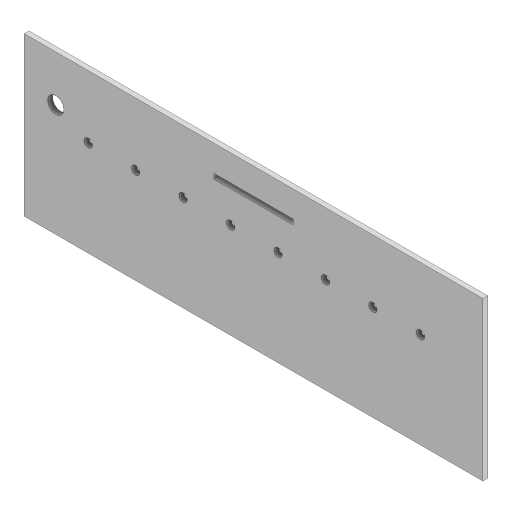
# Autodesk Inventor part: wall_ver.1
Saved by Autodesk Inventor 2024 (Build 280153000, 153)
## iProperties
Created: 2023-11-09
Part Number: wall_ver.1
Material: 一般
Document SubType Name: Modeling
Designer: moonshot
Density: 1 g/cm^3
Appearance: 既定
Author: moonshot
Autodesk Inventor part; units mm, degrees
ref_plane "YZ Plane" through (0, 0, 0) normal (1, 0, 0) x (0, 1, 0)
ref_plane "XZ Plane" through (0, 0, 0) normal (0, 1, 0) x (-1, 0, 0)
ref_plane "XY Plane" through (0, 0, 0) normal (0, 0, 1) x (1, 0, 0)
sketch "スケッチ1" plane through (0, 0, 0) normal (0, 0, 1) x (1, 0, 0)
  line L0 (-145, 50) -> (145, 50)
  line L1 (145, 50) -> (145, -50)
  line L2 (145, -50) -> (-145, -50)
  line L3 (-145, -50) -> (-145, 50)
  line L4 (0, -70) -> (0, 70) projected
  line L5 (-203, 0) -> (203, 0) projected
  circle A0 centre (-104.5, 10.5) radius 2.6
  circle A1 centre (-125, 21) radius 5.1
  circle A2 centre (-74.5, 10.5) radius 2.6
  circle A3 centre (-44.5, 10.5) radius 2.6
  circle A4 centre (-14.5, 10.5) radius 2.6
  circle A5 centre (15.5, 10.5) radius 2.6
  circle A6 centre (45.5, 10.5) radius 2.6
  circle A7 centre (75.5, 10.5) radius 2.6
  circle A8 centre (105.5, 10.5) radius 2.6
  line L6 (-25, 33.5) -> (25, 33.5)
  line L7 (25, 33.5) -> (25, 30.5)
  line L8 (25, 30.5) -> (-25, 30.5)
  line L9 (-25, 30.5) -> (-25, 33.5)
  point P0 (0, 0)
  dimension "d0" = 100
  dimension "d1" = 290
  dimension "d4" = 5.2
  dimension "d5" = 60.5
  dimension "d6" = 40.5
  dimension "d21" = 10.2
  dimension "d22" = 71
  dimension "d23" = 20
  dimension "d26" = 30
  dimension "d31" = 16.5
  dimension "d32" = 50
  dimension "d33" = 3
  constraints: 16 end point, 9 centre point, 4 parallel, 3 horizontal, 2 perpendicular, 17 other
  measures "d0" distance of L2.end L0.start
  measures "d1" distance of L1.end L2.end
  measures "d4" diameter of A0
  measures "d5" distance from line of L2 A0.centre
  measures "d6" distance from line of L3 A0.centre
  measures "d21" diameter of A1
  measures "d22" distance from line of L2 A1.centre
  measures "d23" distance from line of L3 A1.centre
  measures "d26" distance of A0.centre A2.centre
  measures "d31" distance between parallel lines of L6 L0
  measures "d32" distance of L6.start L6.end
  measures "d33" distance of L6.end L7.end
extrude "押し出し1" add sketch "スケッチ1" along normal mid plane 3 contours L0 L4 L6 L9 L8 L5 L3 | L0 L1 L5 L4 L8 L7 L6 | L5 L4 L2 L3 | L5 L1 L2 L4
